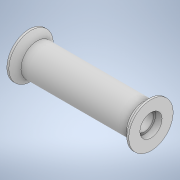
# Autodesk Inventor part: Riiserolle
Saved by Autodesk Inventor 2021 (Build 250183000, 183)
## iProperties
Created: 2024-02-02
Part Number: Riiserolle
Material: Generic
Document SubType Name: Modeling
Designer: Lukas
Density: 1 g/cm^3
Appearance: Default
Author: Lukas
Autodesk Inventor part; units mm, degrees
ref_plane "YZ Plane" through (0, 0, 0) normal (1, 0, 0) x (0, 1, 0)
ref_plane "XZ Plane" through (0, 0, 0) normal (0, 1, 0) x (-1, 0, 0)
ref_plane "XY Plane" through (0, 0, 0) normal (0, 0, 1) x (1, 0, 0)
sketch "Sketch1" plane through (0, 0, 0) normal (0, 0, 1) x (1, 0, 0)
  line L0 (-60.5, 11) -> (-54, 11)
  line L1 (-54, 11) -> (-54, 9)
  line L2 (-54, 9) -> (54, 9)
  line L3 (54, 9) -> (54, 11)
  line L4 (54, 11) -> (60.5, 11)
  line L5 (60.5, 11) -> (60.5, 22)
  line L6 (60.5, 22) -> (58.5, 22)
  line L7 (58.5, 22) -> (52.5, 16)
  line L8 (52.5, 16) -> (-52.5, 16)
  line L9 (-52.5, 16) -> (-58.5, 22)
  line L10 (-58.5, 22) -> (-60.5, 22)
  line L11 (-60.5, 22) -> (-60.5, 11)
  line L12 (-84.7, 0) -> (84.7, 0) projected
  point P0 (0, 0)
  point P1 (0, 16)
  point P2 (0, 9)
  dimension "d0" = 11
  dimension "d1" = 6.5
  dimension "d2" = 9
  dimension "d4" = 105
  dimension "d6" = 2
  dimension "d7" = 16
  dimension "d8" = 22
  constraints: 24 end point, 7 perpendicular, 4 point on line, 2 equal length, 2 midpoint, 2 vertical alignment, 1 horizontal, 1 parallel
  measures "d0" distance from line of point (0, 0) L0
  measures "d1" distance of L0.start L0.end
  measures "d2" distance from line of point (0, 0) L2
  measures "d4" distance of L7.end L8.end
  measures "d6" distance of L9.end L10.end
  measures "d7" distance from line of point (0, 0) L8
  measures "d8" distance from line of point (0, 0) L10
revolve "Revolution1" add sketch "Sketch1" angle 360 about axis through (-10, 0, 0) along (1, 0, 0)
body "Solid1"
